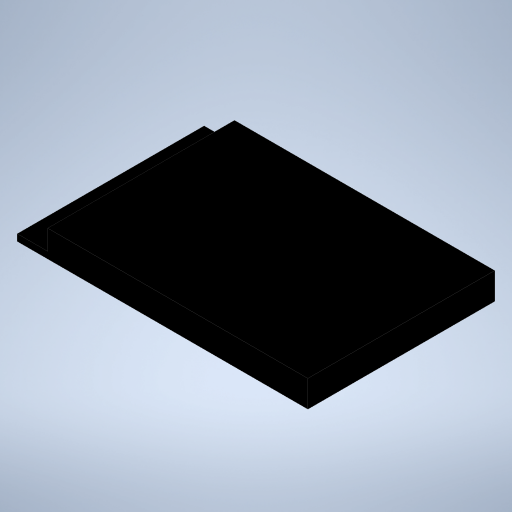
# Autodesk Inventor part: screen
Saved by Autodesk Inventor 2023 (Build 270158000, 158)
## iProperties
Created: 2023-09-25
Part Number: screen
Material: Generic
Document SubType Name: Modeling
Designer: Gage
Density: 1 g/cm^3
Appearance: Default
Author: Gage
Autodesk Inventor part; units mm, degrees
ref_plane "YZ Plane" through (0, 0, 0) normal (1, 0, 0) x (0, 1, 0)
ref_plane "XZ Plane" through (0, 0, 0) normal (0, 1, 0) x (-1, 0, 0)
ref_plane "XY Plane" through (0, 0, 0) normal (0, 0, 1) x (1, 0, 0)
sketch "Sketch1" plane through (0, 0, 0) normal (0, 1, 0) x (-1, 0, 0)
  line L0 (34.8258, -25.0031) -> (-34.8258, -25.0031)
  line L1 (-34.8258, -25.0031) -> (-34.8258, 25.0031)
  line L2 (-34.8258, 25.0031) -> (34.8258, 25.0031)
  line L3 (34.8258, 25.0031) -> (34.8258, -25.0031)
  point P0 (0, 0)
  point P1 (-34.8258, 0)
  point P2 (0, -25.0031)
  dimension "d0" = 69.6516
  dimension "d1" = 50.0063
  constraints: 8 end point, 2 midpoint, 2 parallel, 1 horizontal, 1 horizontal alignment, 1 perpendicular, 1 vertical alignment
  measures "d0" distance of L1.end L2.end
  measures "d1" distance of L0.end L1.end
extrude "Extrusion1" add sketch "Sketch1" along normal blind 5.3578
sketch "Sketch2" plane through (0, 0, 0) normal (0, -1, 0) x (1, 0, 0)
  line L0 (34.8258, 25.0031) -> (34.8258, -25.0031) projected
  line L1 (-34.8258, 25.0031) -> (34.8258, 25.0031) projected
  line L2 (34.8258, -25.0031) -> (-34.8258, -25.0031)
  line L3 (-34.8258, -25.0031) -> (-34.8258, 25.0031)
  line L4 (-34.8258, 25.0031) -> (34.8258, 25.0031)
  line L5 (34.8258, 25.0031) -> (34.8258, -25.0031)
  line L6 (-34.8258, 25.0031) -> (-42.9617, 25.0031)
  line L7 (-42.9617, 25.0031) -> (-42.9617, -25.0031)
  line L8 (-42.9617, -25.0031) -> (-34.8258, -25.0031)
  line L9 (-34.8258, -25.0031) -> (-34.8258, 25.0031)
  point P0 (0, 0)
  dimension "d4" = 8.1359
  constraints: 16 end point, 4 parallel, 2 horizontal, 2 perpendicular, 1 point on line
  measures "d4" distance of L8.end L7.end
extrude "Extrusion2" add sketch "Sketch2" along normal blind 1.7859
body "Solid1"
